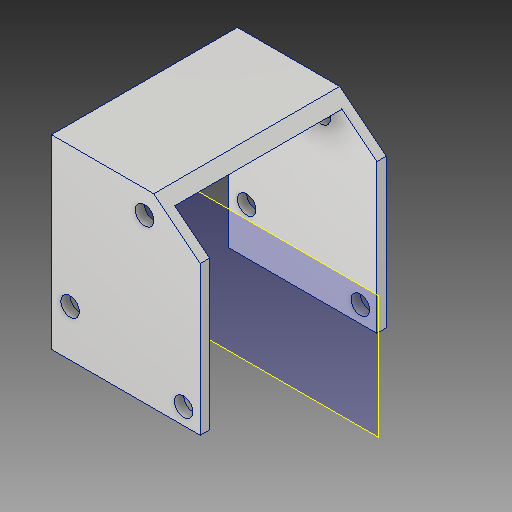
# Autodesk Inventor part: CAR_024_KickerUChannel
Saved by Autodesk Inventor 2018.3 (Build 223284000, 284)
## iProperties
Created: 2020-02-03
Part Number: CAR_024_KickerUChannel
Material: Aluminum 6061
Document SubType Name: Modeling
Designer: user
Mass: 70.0317 g
Surface Area: 183.555 cm^2
Volume: 25.9377 cm^3
Density: 2.7 g/cm^3
Appearance: Aluminum - Flat
Author: user
Autodesk Inventor part; units mm, degrees
ref_plane "YZ Plane" through (0, 0, 0) normal (1, 0, 0) x (0, 1, 0)
ref_plane "XZ Plane" through (0, 0, 0) normal (0, 1, 0) x (-1, 0, 0)
ref_plane "XY Plane" through (0, 0, 0) normal (0, 0, 1) x (1, 0, 0)
sketch "Sketch1" plane through (0, 0, 0) normal (1, 0, 0) x (0, 1, 0)
  line L0 (0, 0) -> (63.5, 0)
  line L1 (63.5, 0) -> (63.5, -63.5)
  line L2 (63.5, -63.5) -> (0, -63.5)
  line L3 (60.325, -3.175) -> (3.175, -3.175)
  line L4 (3.175, -60.325) -> (60.325, -60.325)
  line L5 (60.325, -60.325) -> (60.325, -3.175)
  line L6 (3.175, -3.175) -> (-12.9864, -3.175)
  line L7 (3.175, -60.325) -> (-8.5998, -60.325)
  line L8 (0, -63.5) -> (0, -60.325)
  line L9 (0, -3.175) -> (0, 0)
  dimension "d6" = 63.5
  dimension "d7" = 3.175
  constraints: 20 end point, 4 parallel, 4 perpendicular, 3 horizontal, 2 point on line, 1 other
  measures "d6" distance of L0.end L1.end
  measures "d7" distance between parallel lines of L0 L3
extrude "Extrusion1" add sketch "Sketch1" along normal blind 50.8
ref_plane "Work Plane1" through (0, 0, -31.75) normal (0, 0, -1) x (-1, 0, 0)
sketch "Sketch2" plane through (0, 0, 0) normal (0, 0, 1) x (1, 0, 0)
  line L0 (0, 0) -> (0, 63.5) projected
  line L1 (0, 63.5) -> (50.8, 63.5) projected
  line L2 (0, 0) -> (50.8, 0) projected
  point P0 (6.35, 15.875)
  dimension "d33" = 15.875
  dimension "d34" = 6.35
  measures "d33" distance from line of L2 point (6.35, 15.875)
  measures "d34" distance from line of point (6.35, 15.875) L0
hole "Hole1" at (6.35, 15.875, 0) direction (0, 0, -1) diameter 6.35 end through all
sketch "Sketch4" plane through (0, 0, 0) normal (0, 0, 1) x (1, 0, 0)
  line L0 (50.8, 0) -> (50.8, 63.5) projected
  line L1 (50.8, 63.5) -> (34.925, 63.5)
  line L2 (34.925, 63.5) -> (34.925, 57.15)
  line L3 (50.8, 50.8) -> (50.8, 63.5)
  line L4 (50.8, 50.8) -> (34.925, 63.5)
  point P0 (0, 0)
  dimension "d58" = 15.875
  dimension "d60" = 12.7
  constraints: 8 end point, 1 horizontal, 1 parallel, 1 perpendicular
  measures "d58" distance of L0.end L1.end
  measures "d60" distance from line of L1 L3.start
extrude "Extrusion2" cut sketch "Sketch4" against normal through all
sketch "Sketch3" plane through (0, 0, 0) normal (0, 0, 1) x (1, 0, 0)
  circle A0 centre (6.35, 15.875) radius 3.175 construction
  line L0 (0, 0) -> (0, 63.5) construction
  line L1 (0, 0) -> (50.8, 0) construction
  line L2 (50.8, 50.8) -> (50.8, 0) construction
  line L3 (0, 63.5) -> (34.925, 63.5) construction
  line L4 (9.8817, -6.9679) -> (-8.7166, 33.4041) construction
  line L5 (-8.7166, 33.4041) -> (298.3815, 174.8763) construction
  line L6 (298.3815, 174.8763) -> (316.9799, 134.5042) construction
  line L7 (316.9799, 134.5042) -> (9.8817, -6.9679) construction
  line L8 (0, 60.325) -> (50.8, 60.325) construction
  line L9 (50.8, 50.8) -> (34.925, 63.5) projected
  point P0 (45.1543, 5.6457)
  point P1 (31.795, 55.5625)
  point P2 (288.925, 146.05)
  dimension "d36" = 6.35
  dimension "d38" = 5.6457
  dimension "d41" = 44.45
  dimension "d43" = 3.302
  dimension "d44" = 3.175
  dimension "d46" = 22.225
  dimension "d49" = 22.225
  dimension "d50" = 20.6502
  dimension "d52" = 130.175
  dimension "d53" = 4.7625
  dimension "d54" = 282.575
  dimension "d55" = 24.734
  dimension "d56" = 338.1178
  dimension "d57" = 5.6457
  constraints: 8 end point, 2 parallel, 1 perpendicular
  measures "d36" distance from line of L4 A0.centre
  measures "d38" distance from line of L2 point (45.154, 5.646)
  measures "d41" distance of L4.start L4.end
  measures "d43" distance from line of L7 point (45.154, 5.646)
  measures "d44" distance from line of L5 point (31.795, 55.562)
  measures "d46" distance from line of L5 A0.centre
  measures "d49" distance from line of L5 point (288.925, 146.05)
  measures "d50" distance from line of L6 point (288.925, 146.05)
  measures "d52" vertical distance of point (288.925, 146.05) A0.centre
  measures "d53" distance from line of point (31.795, 55.562) L8
  measures "d54" horizontal distance of point (288.925, 146.05) A0.centre
  measures "d55" angle of L8 L5
  measures "d56" distance of L6.end L4.start
  measures "d57" distance from line of point (45.154, 5.646) L1
hole "Hole2" at (45.1543, 5.6457, 0) at (31.795, 55.5625, 0) direction (0, 0, -1) diameter 6.35 end through all
equation "\"d57\" = d38"
body "Solid1"
